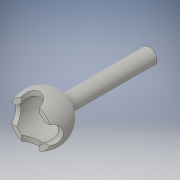
# Autodesk Inventor part: RTS Caster
Saved by Autodesk Inventor 2016 (Build 200138000, 138)
## iProperties
Created: 2016-10-20
Part Number: RTS Caster
Material: Generic
Document SubType Name: Modeling
Designer: sullir
Density: 1 g/cm^3
Appearance: Default
Author: sullir
Autodesk Inventor part; units mm, degrees
ref_plane "YZ Plane" through (0, 0, 0) normal (1, 0, 0) x (0, 1, 0)
ref_plane "XZ Plane" through (0, 0, 0) normal (0, 1, 0) x (-1, 0, 0)
sketch "Sketch1" plane through (0, 0, 0) normal (0, 0, 1) x (1, 0, 0)
  point P0 (0, 0)
sketch "Sketch2" plane through (0, 0, 0) normal (0, 0, 1) x (1, 0, 0)
  circle A0 centre (0, 0) radius 3.81
  dimension "d0" = 7.62
  constraints: 1 centre point, 1 coincident
  measures "d0" diameter of A0
extrude "Extrusion1" add sketch "Sketch2" along normal blind 29.5148
sketch "Sketch3" plane through (0, 0, 29.5148) normal (0, 0, 1) x (1, 0, 0)
  arc A0 (0, -11.8745) -> (0, 11.8745) centre (0, 0) ccw
  line L0 (0, 11.8745) -> (0, -11.8745)
  dimension "d3" = 23.749
  constraints: 2 end point, 2 point on circle, 1 centre point, 1 coincident
  measures "d3" diameter of A0
revolve "Revolution1" add sketch "Sketch3" angle 360 about axis through (0, 11.8745, 29.5148) along (0, -1, 0)
sketch "Sketch4" plane through (0, 0, 0) normal (1, 0, 0) x (0, 1, 0)
  point P0 (0, 0)
sketch "Sketch6" plane through (0, 0, 0) normal (0, 1, 0) x (-1, 0, 0)
  arc A0 (0, 39.8015) -> (0, 20.9955) centre (0, 30.3985) ccw
  line L0 (0, 20.9955) -> (0, 39.8015)
  point P0 (0, 0)
  constraints: 2 end point, 2 point on circle, 1 centre point, 1 vertical
revolve "Revolution3" cut sketch "Sketch6" angle 360 about axis through (0, 0, 20.9955) along (0, 0, 1)
ref_plane "Work Plane1" through (0, 0, 34.925) normal (0, 0, 1) x (1, 0, 0)
sketch "Sketch5" plane through (0, 0, 34.925) normal (0, 0, 1) x (1, 0, 0)
  circle A0 centre (0, 0) radius 23.6946
  line L0 (-23.6946, 0) -> (23.6946, 0)
  constraints: 2 end point, 2 point on circle, 1 centre point, 1 coincident, 1 horizontal
revolve "Revolution2" cut sketch "Sketch5" angle 180 about axis through (-23.6946, 0, 34.925) along (-1, 0, 0) picked at (3.7054, -11.0554) contours A0 L0
sketch "Sketch7" plane through (0, 0, 0) normal (1, 0, 0) x (0, 1, 0)
  point P0 (0, 0)
sketch "Sketch8" plane through (0, 0, 0) normal (1, 0, 0) x (0, 1, 0)
  line L0 (8.2418, 34.925) -> (-8.2418, 34.925) projected
  circle A0 centre (0, 34.925) radius 4.5339
  point P0 (0, 0)
  dimension "d8" = 9.0678
  constraints: 1 centre point, 1 midpoint
  measures "d8" diameter of A0
extrude "Extrusion2" cut sketch "Sketch8" along normal mid plane 48.5648
sketch "Sketch9" plane through (0, 0, 0) normal (0, 1, 0) x (-1, 0, 0)
  line L0 (-9.5487, 34.925) -> (9.5487, 34.925) projected
  circle A0 centre (0, 34.925) radius 4.5339
  point P0 (0, 0)
  dimension "d11" = 9.0678
  constraints: 1 centre point, 1 midpoint
  measures "d11" diameter of A0
extrude "Extrusion3" cut sketch "Sketch9" along normal mid plane 48.5648
sketch "Sketch10" plane through (0, 0, 0) normal (0, 0, -1) x (-1, 0, 0)
  circle A0 centre (0, 0) radius 3.81
  constraints: 1 centre point, 1 coincident
extrude "Extrusion4" add sketch "Sketch10" along normal blind 25.4
sketch "Sketch11" plane through (0, 0, -25.4) normal (0, 0, -1) x (-1, 0, 0)
  circle A0 centre (0, 0) radius 3.81
  constraints: 1 centre point, 1 coincident
extrude "Extrusion5" cut sketch "Sketch11" against normal blind 25.4
sketch "Sketch12" plane through (0, 0, 0) normal (0, 0, -1) x (-1, 0, 0)
  circle A0 centre (0, 0) radius 3.81
  constraints: 1 centre point, 1 coincident
extrude "Extrusion6" add sketch "Sketch12" along normal blind 20.32
sketch "Sketch13" plane through (0, 0, -20.32) normal (0, 0, -1) x (-1, 0, 0)
  circle A0 centre (0, 0) radius 3.81
  constraints: 1 centre point, 1 coincident
extrude "Extrusion7" add sketch "Sketch13" along normal blind 2.54
sketch "Sketch14" plane through (0, 0, -22.86) normal (0, 0, -1) x (-1, 0, 0)
  circle A0 centre (0, 0) radius 3.81
  constraints: 1 centre point, 1 coincident
extrude "Extrusion8" add sketch "Sketch14" along normal blind 0.762
sketch "Sketch15" plane through (0, 0, -23.622) normal (0, 0, -1) x (-1, 0, 0)
  circle A0 centre (0, 0) radius 3.81
  constraints: 1 centre point, 1 coincident
extrude "Extrusion9" add sketch "Sketch15" along normal blind 0.762
body "Solid1"
